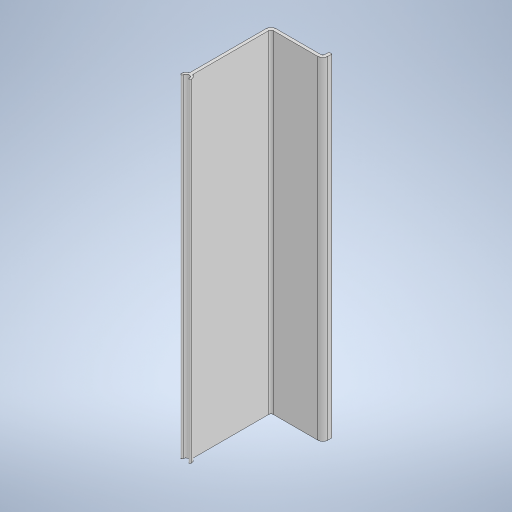
# Autodesk Inventor part: Light Cover
Saved by Autodesk Inventor 2023.4 (Build 274418000, 418)
## iProperties
Created: 2024-07-24
Part Number: Light Cover
Material: Generic
Document SubType Name: Modeling
Designer: Nathan Cai
Density: 1 g/cm^3
Appearance: Default
Author: Nathan Cai
Autodesk Inventor part; units mm, degrees
ref_plane "YZ Plane" through (0, 0, 0) normal (1, 0, 0) x (0, 1, 0)
ref_plane "XZ Plane" through (0, 0, 0) normal (0, 1, 0) x (-1, 0, 0)
ref_plane "XY Plane" through (0, 0, 0) normal (0, 0, 1) x (1, 0, 0)
sketch "Sketch1" plane through (0, 0, 0) normal (0, 1, 0) x (-1, 0, 0)
  line L0 (0, 0) -> (-1.5, 0)
  line L1 (-1.5, 0) -> (-1.5, 41)
  line L2 (-1.5, 41) -> (0, 41) construction
  line L3 (0, 41) -> (0, 0)
  line L4 (0, 0) -> (-27, 0)
  line L5 (-27, 0) -> (-27, 1.5)
  line L6 (-27, 1.5) -> (0, 1.5)
  line L7 (0, 1.5) -> (0, 0)
  line L8 (-27, 1.5) -> (-25.5, 1.5)
  line L9 (-25.5, 1.5) -> (-25.5, -3)
  line L10 (-25.5, -3) -> (-27, -3)
  line L11 (-27, -3) -> (-27, 1.5)
  arc A0 (-2.25, 42.5) -> (0.75, 42.5) centre (-0.75, 42.5) ccw
  line L12 (-0.75, 41) -> (-0.75, 42.5) construction
  line L13 (-0.75, 42.5) -> (0.75, 42.5) construction
  arc A1 (1.75, 42.5) -> (0.75, 42.5) centre (1.25, 42.5) ccw
  arc A2 (-3.25, 42.5) -> (1.75, 42.5) centre (-0.75, 42.5) ccw
  arc A3 (-2.25, 42.5) -> (-3.25, 42.5) centre (-2.75, 42.5) ccw
  point P0 (-0.75, 41)
  point P1 (-25.5, 0)
  point P2 (0, 40.1152)
  point P3 (-1.5, 40.1152)
  point P4 (-1.5, 1.5)
  dimension "d0" = 1.5
  dimension "d1" = 41
  dimension "d2" = 27
  dimension "d3" = 1.5
  dimension "d4" = 1.5
  dimension "d5" = 4.5
  dimension "d6" = 3
  dimension "d7" = 1
  constraints: 28 end point, 9 point on circle, 6 parallel, 4 centre point, 4 horizontal, 4 perpendicular, 3 tangent, 2 midpoint, 2 point on line, 1 coincident, 1 symmetric about line, 1 other
  measures "d0" distance of L1.end L2.end
  measures "d1" distance of L0.end L1.end
  measures "d2" distance of L5.end L6.end
  measures "d3" distance of L4.end L5.end
  measures "d4" distance of L9.end L10.end
  measures "d5" distance of L8.end L9.end
  measures "d6" diameter of A0
  measures "d7" diameter of A1
extrude "Extrusion1" add sketch "Sketch1" along normal blind 163.5125
fillet "Fillet1" radius 2.5 2 edges at (0, 81.7562, 0) (27, 81.7562, 1.5)
fillet "Fillet2" radius 1 2 edges at (1.5, 81.7562, 1.5) (25.5, 81.7562, 0)
fillet "Fillet3" radius 0.5 2 edges at (0, 81.7562, 40.1152) (1.5, 81.7562, 40.1152)
body "Solid1"
